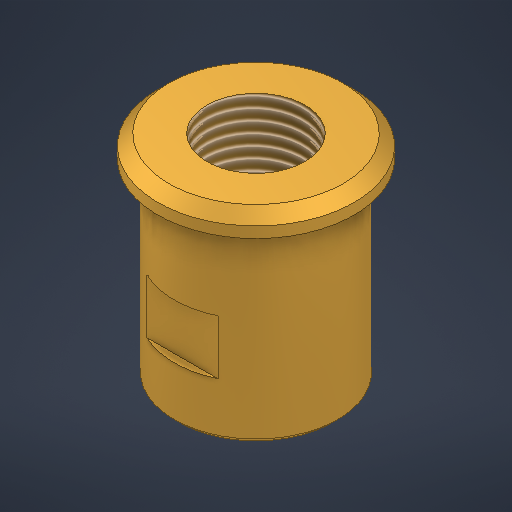
# Autodesk Inventor part: Part2
Saved by Autodesk Inventor 2026.2 (Build 302298010, 298A)
## iProperties
Created: 2026-03-22
Part Number: Part2
Material: Generic
Document SubType Name: Modeling
Designer: Mlinč
Density: 1 g/cm^3
Appearance: Default
Author: Mlinč
Autodesk Inventor part; units mm, degrees
ref_plane "YZ Plane" through (0, 0, 0) normal (1, 0, 0) x (0, 1, 0)
ref_plane "XZ Plane" through (0, 0, 0) normal (0, 1, 0) x (-1, 0, 0)
sketch "Sketch1" plane through (0, 0, 0) normal (0, 0, 1) x (1, 0, 0)
  line L0 (-9, 0) -> (-15, 0)
  line L1 (-15, 0) -> (-15, 35)
  line L2 (-15, 35) -> (-18, 35)
  line L3 (-18, 35) -> (-18, 37)
  line L4 (-18, 37) -> (-16, 39)
  line L5 (-16, 39) -> (-9, 39)
  line L6 (-9, 39) -> (-9, 0)
  line L7 (0, 39) -> (0, 0)
  dimension "d0" = 18
  dimension "d1" = 30
  dimension "d2" = 36
  dimension "d3" = 32
  dimension "d4" = 2
  dimension "d5" = 2
  dimension "d6" = 39
  constraints: 16 end point, 4 perpendicular, 2 parallel, 1 horizontal, 1 horizontal alignment, 1 vertical
  measures "d0" diameter of L6 L7
  measures "d1" diameter of L1 L7
  measures "d2" diameter of L3 L7
  measures "d3" diameter of L4.end L7
  measures "d4" distance from line of L3.end L5
  measures "d5" distance of L2.end L3.end
  measures "d6" distance between parallel lines of L0 L5
revolve "Revolution1" add sketch "Sketch1" angle 360 about axis through (0, 39, 0) along (0, -1, 0)
chamfer "Chamfer1" distance 1 angle 45 1 edges at (15, 0, 0)
thread "Thread1" size "TR20x2" class "7H" standard "ISO Metric Trapezoidal Threads" full length
ref_plane "Work Plane2" through (0, 17.5, 15) normal (0, 0, 1) x (1, 0, 0)
sketch "Sketch3" plane through (0, 17.5, 15) normal (0, 0, 1) x (1, 0, 0)
  line L0 (12.5, -7.5) -> (-12.5, -7.5)
  line L1 (-12.5, -7.5) -> (-12.5, 2.5)
  line L2 (-12.5, 2.5) -> (12.5, 2.5)
  line L3 (12.5, 2.5) -> (12.5, -7.5)
  line L4 (12.5, -7.5) -> (-12.5, 2.5) construction
  line L5 (-12.5, -7.5) -> (12.5, 2.5) construction
  point P0 (0, -17.5)
  point P1 (0, -2.5)
  dimension "d16" = 25
  dimension "d17" = 10
  dimension "d18" = 15
  constraints: 12 end point, 2 midpoint, 2 parallel, 1 horizontal, 1 perpendicular, 1 vertical alignment
  measures "d16" distance of L1.end L2.end
  measures "d17" distance of L0.end L1.end
  measures "d18" distance of point (0, -17.5) point (0, -2.5)
extrude "Extrusion1" cut sketch "Sketch3" against normal blind 1.5
body "Solid1"
